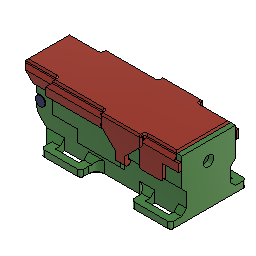
ratcase 1 v10 (Autodesk Fusion 360 design; units mm, degrees)
Autodesk Fusion 360 part; units mm, degrees
sketch "Sketch1" plane through (0, 0, 0) normal (0, 0, 1) x (1, 0, 0)
  line L0 (38, -11) -> (-38, -11)
  line L1 (-38, -11) -> (-38, 11)
  line L2 (-38, 11) -> (38, 11)
  line L3 (38, 11) -> (38, -11)
  line L4 (38, -11) -> (-38, 11) construction
  line L5 (-38, -11) -> (38, 11) construction
  line L6 (41, -14) -> (-41, -14)
  line L7 (-41, -14) -> (-41, 14)
  line L8 (-41, 14) -> (41, 14)
  line L9 (41, 14) -> (41, -14)
  dimension "d1" = 76
  dimension "d2" = 22
  dimension "d3" = -3
  constraint horizontal L0
  constraint perpendicular L0 L1
  constraint parallel L0 L2
  constraint parallel L1 L3
  constraint coincident L4 origin
  constraint coincident L5 origin
  measures "d1" distance of L1.end L2.end
  measures "d2" distance of L0.end L1.end
extrude "Extrude1" add sketch "Sketch1" along normal blind 20 makes body 1
sketch "Sketch15" plane through (0, 0, 20) normal (0, 0, 1) x (-1, 0, 0)
  line L0 (38, -11) -> (-38, -11)
  line L1 (-38, -11) -> (-38, 11)
  line L2 (-38, 11) -> (38, 11)
  line L3 (38, 11) -> (38, -11)
  line L4 (-41, -14) -> (41, -14)
  line L5 (41, -14) -> (41, 14)
  line L6 (41, 14) -> (-41, 14)
  line L7 (-41, 14) -> (-41, -14)
  line L8 (38, -11) -> (39, -11)
  line L9 (39, -11) -> (39, -7)
  line L10 (39, -7) -> (38, -7)
  line L11 (38, -7) -> (38, -11)
  line L12 (-38, 11) -> (-39, 11)
  line L13 (-39, 11) -> (-39, 7)
  line L14 (-39, 7) -> (-38, 7)
  line L15 (-38, 7) -> (-38, 11)
  dimension "d64" = 1
  dimension "d65" = 4
  dimension "d66" = 1
  dimension "d67" = 4
  constraint horizontal L8
  constraint vertical L9
  constraint horizontal L10
  constraint vertical L11
  constraint coincident L0.start L3.end
  constraint horizontal L12
  constraint vertical L13
  constraint horizontal L14
  constraint vertical L15
  constraint coincident L1.end L2.start
  measures "d64" distance of L1.end L12.end
  measures "d65" distance of L12.end L13.end
  measures "d66" distance of L9.end L10.end
  measures "d67" distance of L8.end L9.end
extrude "Extrude15" cut sketch "Sketch15" against normal blind 59 contours L3 L8 L9 L10 L11 | L1 L12 L13 L14 L15 bodies 1
sketch "Sketch2" plane through (0, 0, 0) normal (0, 0, -1) x (1, 0, 0)
  line L0 (38, -11) -> (-39, -11)
  line L1 (-38, -7) -> (-38, 11)
  line L2 (-38, 11) -> (39, 11)
  line L3 (38, 7) -> (38, -11)
  line L4 (-41, -14) -> (41, -14)
  line L5 (41, -14) -> (41, 14)
  line L6 (41, 14) -> (-41, 14)
  line L7 (-41, 14) -> (-41, -14)
  line L8 (-41, 14) -> (41, 14)
  line L9 (41, 14) -> (41, -14)
  line L10 (41, -14) -> (-41, -14)
  line L11 (-41, -14) -> (-41, 14)
  line L12 (39, 7) -> (38, 7)
  line L13 (-39, -7) -> (-38, -7)
  line L14 (39, 11) -> (39, 7)
  line L15 (-39, -11) -> (-39, -7)
  constraint horizontal L8
  constraint vertical L9
  constraint horizontal L10
  constraint vertical L11
  constraint coincident L4.end L5.start
  constraint coincident L6.end L7.start
extrude "Extrude2" add sketch "Sketch2" along normal blind 3 contours L0 L1 L2 L3 L12 L13 L14 L15 | L4 L5 L6 L7 L8 L9 L10 L11 bodies 1
sketch "Sketch3" plane through (0, 0, 20) normal (0, 0, 1) x (-1, 0, 0)
  line L0 (-38, -11) -> (-38, 7)
  line L1 (-41, -14) -> (41, -14)
  line L2 (41, -14) -> (41, 14)
  line L3 (41, 14) -> (-41, 14)
  line L4 (-41, 14) -> (-41, -14)
  line L5 (38, -14) -> (-2, -14)
  line L6 (-2, -14) -> (-2, 14)
  line L7 (-2, 14) -> (38, 14)
  line L8 (38, 14) -> (38, -14)
  line L9 (38, -14) -> (-2, 14) construction
  line L10 (-2, -14) -> (38, 14) construction
  line L11 (18, 0) -> (0, 0) construction
  line L12 (-31, 14) -> (-7, 14)
  line L13 (-7, 14) -> (-7, -14)
  line L14 (-7, -14) -> (-31, -14)
  line L15 (-31, -14) -> (-31, 14)
  line L16 (-31, 14) -> (-7, -14) construction
  line L17 (-7, 14) -> (-31, -14) construction
  line L18 (0, 0) -> (-19, 0) construction
  line L19 (41, -17) -> (-41, -17)
  line L20 (-41, -17) -> (-41, 17)
  line L21 (-41, 17) -> (41, 17)
  line L22 (41, 17) -> (41, -17)
  line L23 (-38, 7) -> (-39, 7)
  line L24 (-39, 11) -> (38, 11)
  line L25 (38, 11) -> (38, -7)
  line L26 (38, -7) -> (39, -7)
  line L27 (39, -7) -> (39, -11)
  line L28 (39, -11) -> (-38, -11)
  line L29 (-39, 7) -> (-39, 11)
  point P0 (18, 0)
  point P1 (-19, 0)
  dimension "d8" = 28
  dimension "d9" = 40
  dimension "d10" = 24
  dimension "d13" = 3
  dimension "d14" = 3
  dimension "d68" = 5
  constraint horizontal L5
  constraint perpendicular L5 L6
  constraint parallel L5 L7
  constraint parallel L6 L8
  constraint coincident L9 P0
  constraint coincident L10 P0
  constraint coincident P0 L11.start
  constraint coincident L11.end L18.start
  constraint horizontal L11
  constraint horizontal L12
  constraint perpendicular L12 L13
  constraint parallel L12 L14
  constraint parallel L13 L15
  constraint coincident L16 P1
  constraint coincident L17 P1
  constraint coincident P1 L18.end
  constraint parallel L11 L18
  constraint collinear L5 L14
  constraint horizontal L19
  constraint vertical L20
  constraint horizontal L21
  constraint vertical L22
  constraint collinear L2 L22
  constraint collinear L4 L20
  constraint collinear L8 L25
  measures "d8" distance of L5.start L7.end
  measures "d9" distance of L6.end L7.end
  measures "d10" distance of L12.start L12.end
  measures "d13" distance of L5 L19
  measures "d14" distance of L7 L21
  measures "d68" distance of L6 L13
extrude "Extrude3" add sketch "Sketch3" along normal blind 10 separate body contours L0 L1 L3 L4 L15 L20 L23 L24 L28 L29 | L1 L5 L14 L19 L20 L22 | L1 L6 L13 L28 | L3 L7 L12 L20 L21 L22 | L3 L6 L13 L24 | L1 L2 L3 L8 L22 L25 L26 L27 L28 makes body 2
sketch "Sketch10" plane through (41, 0, 0) normal (1, 0, 0) x (0, 1, 0)
  line L0 (14, -3) -> (14, 20)
  line L1 (14, 20) -> (-14, 20)
  line L2 (-14, 20) -> (-14, -3)
  line L3 (-14, -3) -> (14, -3)
  line L4 (-14, 20) -> (-17, 20)
  line L5 (-17, 20) -> (-17, 17)
  line L6 (-17, 17) -> (-14, 17)
  line L7 (-14, 17) -> (-14, 20)
  line L8 (14, 20) -> (17, 20)
  line L9 (17, 20) -> (17, 17)
  line L10 (17, 17) -> (14, 17)
  line L11 (14, 17) -> (14, 20)
  constraint horizontal L4
  constraint vertical L5
  constraint horizontal L6
  constraint vertical L7
  constraint coincident L1.end L2.start
  constraint horizontal L8
  constraint vertical L9
  constraint horizontal L10
  constraint vertical L11
  constraint coincident L0.end L1.start
extrude "Extrude10" add sketch "Sketch10" against normal up to surface (82 mm away) contours L0 L8 L9 L10 L11 | L2 L4 L5 L6 L7 bodies 1 2
sketch "Sketch4" plane through (0, 0, 20) normal (0, 0, 1) x (-1, 0, 0)
  line L0 (-2, 11) -> (38, 11)
  line L1 (22, -14) -> (22, 14)
  line L2 (1, -14) -> (1, 14)
  line L3 (38, -11) -> (38, -14)
  line L4 (38, 11) -> (38, 14)
  line L5 (-2, 14) -> (-2, 11)
  line L6 (38, 14) -> (-2, 14)
  line L7 (22, -14) -> (1, -14)
  line L8 (1, 14) -> (22, 14)
  line L9 (-2, -14) -> (-2, -11)
  dimension "d18" = 21
  dimension "d158" = 3
  constraint perpendicular L0 L1
  measures "d18" distance of L1 L2
  measures "d158" distance of L2 L9
extrude "Extrude4" cut sketch "Sketch4" against normal blind 7.5 contours L0 L1 L2 L6 L8 | L0 L1 L2 L7 bodies 1
sketch "Sketch5" plane through (0, -14, 0) normal (0, -1, 0) x (1, 0, 0)
  line L0 (-41, 17) -> (-41, -3)
  line L1 (-41, -3) -> (41, -3)
  line L2 (41, -3) -> (41, 17)
  line L3 (-1, 12.5) -> (-22, 12.5)
  line L4 (-25, 20) -> (-25, 9.5)
  line L5 (-25, 9.5) -> (2, 9.5)
  line L6 (2, 9.5) -> (2, 20)
  line L7 (-25, 20) -> (2, 20)
  line L8 (-22, 17) -> (-41, 17)
  line L9 (41, 17) -> (-1, 17)
  line L10 (-1, 17) -> (-1, 12.5)
  line L11 (-22, 12.5) -> (-22, 17)
  dimension "d22" = 3
  dimension "d159" = 3
  dimension "d160" = 3
  constraint perpendicular L0 L5
  constraint vertical L4
  measures "d22" distance of L3 L5
  measures "d159" distance of L4 L11
  measures "d160" distance of L6 L10
extrude "Extrude5" add sketch "Sketch5" along normal blind 3 contours L3 L4 L5 L6 L8 L9 L10 L11 | L3 L4 L6 L7 L8 L9 L10 L11 bodies 1
sketch "Sketch16" plane through (0, 14, 0) normal (0, 1, 0) x (-1, 0, 0)
  line L0 (1, 17) -> (-41, 17)
  line L1 (-41, 17) -> (-41, -3)
  line L2 (-41, -3) -> (41, -3)
  line L3 (41, -3) -> (41, 17)
  line L4 (-2, 17) -> (25, 17)
  line L5 (25, 17) -> (25, 9.5)
  line L6 (25, 9.5) -> (-2, 9.5)
  line L7 (-2, 9.5) -> (-2, 17)
  line L8 (22, 12.5) -> (1, 12.5)
  line L9 (22, 17) -> (22, 12.5)
  line L10 (22, 12.5) -> (1, 12.5)
  line L11 (1, 12.5) -> (1, 17)
  line L12 (41, 17) -> (22, 17)
  dimension "d60" = 3
  dimension "d69" = 3
  dimension "d70" = 3
  constraint horizontal L4
  constraint vertical L5
  constraint horizontal L6
  constraint vertical L7
  constraint coincident L0 L4.start
  measures "d60" distance of L6 L8
  measures "d69" distance of L7 L11
  measures "d70" distance of L5 L9
extrude "Extrude16" add sketch "Sketch16" along normal up to surface (3 mm away) contours L0 L4 L5 L6 L7 L8 L9 L10 L11 L12 | L4 L8 L9 L10 L11 bodies 1
sketch "Sketch7" plane through (41, 0, 0) normal (1, 0, 0) x (0, 1, 0)
  line L0 (14, -3) -> (14, 17)
  line L1 (17, 17) -> (17, 30)
  line L2 (17, 30) -> (-17, 30)
  line L3 (-14, 17) -> (-14, -3)
  line L4 (-14, -3) -> (14, -3)
  circle A0 centre (0, 24) radius 3.25
  line L5 (14, 17) -> (17, 17)
  line L6 (-17, 30) -> (-17, 17)
  line L7 (-17, 17) -> (-14, 17)
  dimension "d28" = 6.5
  dimension "d29" = 6
  measures "d28" diameter of A0
  measures "d29" distance of L2 A0.centre
extrude "Extrude7" cut sketch "Sketch7" against normal blind 6 contours A0 bodies 1
sketch "Sketch8" plane through (0, 0, 30) normal (0, 0, 1) x (-1, 0, 0)
  line L0 (-7, -14) -> (-31, -14)
  line L1 (-31, -14) -> (-31, -11)
  line L2 (-31, 14) -> (-7, 14)
  line L3 (38, 14) -> (38, -7)
  line L4 (41, 17) -> (-41, 17)
  line L5 (-41, 17) -> (-41, -17)
  line L6 (-41, -17) -> (41, -17)
  line L7 (41, -17) -> (41, 17)
  line L8 (-7, 11) -> (-4, 11)
  line L9 (-4, 11) -> (-4, 14)
  line L10 (-4, 14) -> (-7, 14)
  line L11 (-7, 14) -> (-7, 11)
  line L12 (-7, 14) -> (-7, 11)
  line L13 (-2, 11) -> (-2, 14)
  line L14 (-2, 14) -> (38, 14)
  line L15 (38, -14) -> (-2, -14)
  line L16 (-38, 7) -> (-39, 7)
  line L17 (-39, 7) -> (-39, 11)
  line L18 (-39, 11) -> (-31, 11)
  line L19 (-31, 11) -> (-31, 14)
  line L20 (-7, 11) -> (-2, 11)
  line L21 (38, -7) -> (39, -7)
  line L22 (39, -7) -> (39, -11)
  line L23 (39, -11) -> (38, -11)
  line L24 (38, -11) -> (38, -14)
  line L25 (-2, -14) -> (-2, -11)
  line L26 (-2, -11) -> (-7, -11)
  line L27 (-7, -11) -> (-7, -14)
  line L28 (-31, -11) -> (-38, -11)
  line L29 (-38, -11) -> (-38, 7)
  dimension "d71" = 3
  constraint horizontal L8
  constraint vertical L9
  constraint horizontal L10
  constraint vertical L11
  constraint coincident L2.end L10.end
  measures "d71" distance of L9.end L2.end
extrude "Extrude8" cut sketch "Sketch8" against normal up to surface (10 mm away) contours L8 L9 L10 L11 L12 L20 bodies 1
sketch "Sketch9" plane through (0, 0, 30) normal (0, 0, 1) x (-1, 0, 0)
  line L0 (38, 14) -> (38, -7)
  line L1 (-7, -14) -> (-31, -14)
  line L2 (-31, -14) -> (-31, -11)
  line L3 (-31, 14) -> (-4, 14)
  line L4 (41, 17) -> (-41, 17)
  line L5 (-41, 17) -> (-41, -17)
  line L6 (-41, -17) -> (41, -17)
  line L7 (41, -17) -> (41, 17)
  line L8 (-27.5, 14) -> (-19.5, 14)
  line L9 (-19.5, 14) -> (-19.5, 15)
  line L10 (-19.5, 15) -> (-27.5, 15)
  line L11 (-27.5, 15) -> (-27.5, 14)
  line L12 (-2, 11) -> (-2, 14)
  line L13 (-2, 14) -> (38, 14)
  line L14 (38, -14) -> (-2, -14)
  line L15 (-4, 14) -> (-4, 11)
  line L16 (-4, 11) -> (-2, 11)
  line L17 (38, -7) -> (39, -7)
  line L18 (39, -7) -> (39, -11)
  line L19 (39, -11) -> (38, -11)
  line L20 (38, -11) -> (38, -14)
  line L21 (-2, -14) -> (-2, -11)
  line L22 (-2, -11) -> (-7, -11)
  line L23 (-7, -11) -> (-7, -14)
  line L24 (-31, -11) -> (-38, -11)
  line L25 (-38, -11) -> (-38, 7)
  line L26 (-38, 7) -> (-39, 7)
  line L27 (-39, 7) -> (-39, 11)
  line L28 (-39, 11) -> (-31, 11)
  line L29 (-31, 11) -> (-31, 14)
  dimension "d35" = 8
  dimension "d36" = 1
  dimension "d72" = 3.5
  constraint horizontal L8
  constraint vertical L9
  constraint horizontal L10
  constraint vertical L11
  constraint coincident L3 L8.start
  measures "d35" distance of L9.end L10.end
  measures "d36" distance of L8.end L9.end
  measures "d72" distance of L11 L29
extrude "Extrude9" cut sketch "Sketch9" against normal up to surface (10 mm away) contours L3 L8 L9 L10 L11 bodies 1
sketch "Sketch11" plane through (41, 0, 0) normal (1, 0, 0) x (0, 1, 0)
  circle A0 centre (0, 24) radius 3.25
  line L0 (14, 17) -> (17, 17)
  line L1 (17, 17) -> (17, 30)
  line L2 (17, 30) -> (-17, 30)
  line L3 (-17, 30) -> (-17, 17)
  line L4 (-17, 17) -> (-14, 17)
  line L5 (-14, 17) -> (-14, -3)
  line L6 (-14, -3) -> (14, -3)
  line L7 (14, -3) -> (14, 17)
  line L8 (-17, 30) -> (17, 30)
  line L9 (17, 30) -> (17, 35)
  line L10 (17, 35) -> (-17, 35)
  line L11 (-17, 35) -> (-17, 30)
  dimension "d45" = 5
  constraint horizontal L8
  constraint vertical L9
  constraint horizontal L10
  constraint vertical L11
  constraint coincident L2.end L3.start
  measures "d45" distance of L2.end L10.end
extrude "Extrude11" add sketch "Sketch11" against normal up to surface (3 mm away) contours L2 L8 L9 L10 L11 bodies 1
sketch "Sketch12" plane through (0, 17, 0) normal (0, 1, 0) x (-1, 0, 0)
  line L0 (41, 17) -> (41, 30)
  line L1 (41, 30) -> (-38, 30)
  line L2 (-41, 35) -> (-41, 17)
  line L3 (-41, 17) -> (-2, 17)
  line L4 (-38, 30) -> (-39, 30)
  line L5 (-39, 30) -> (-39, 32.5)
  line L6 (-39, 32.5) -> (-38, 33.5)
  line L7 (-2, 17) -> (-2, 9.5)
  line L8 (-2, 9.5) -> (25, 9.5)
  line L9 (25, 9.5) -> (25, 17)
  line L10 (25, 17) -> (41, 17)
  line L11 (-38, 30) -> (-38, 35)
  line L12 (-38, 35) -> (-41, 35)
  line L13 (-38, 30) -> (-38, 33.5)
  constraint coincident L1.end L4.start
  constraint perpendicular L1 L5
extrude "Extrude12" cut sketch "Sketch12" against normal blind 34 contours L4 L5 L6 L11 L13 bodies 1
sketch "Sketch13" plane through (0, -17, 0) normal (0, -1, 0) x (1, 0, 0)
  line L0 (39, 30) -> (-41, 30)
  line L1 (-41, 30) -> (-41, 17)
  line L2 (-25, 9.5) -> (2, 9.5)
  line L3 (2, 9.5) -> (2, 17)
  line L4 (41, 17) -> (41, 35)
  line L5 (38, 30) -> (39, 30)
  line L6 (39, 30) -> (39, 33.5)
  line L7 (39, 33.5) -> (38, 33.5)
  line L8 (38, 33.5) -> (38, 30)
  line L9 (38, 33.5) -> (39, 32.5)
  line L10 (39, 32.5) -> (39, 30)
  line L11 (-41, 17) -> (-25, 17)
  line L12 (41, 35) -> (38, 35)
  line L13 (38, 35) -> (38, 33.5)
  line L14 (39, 32.5) -> (39, 30)
  line L15 (-25, 17) -> (-25, 9.5)
  line L16 (2, 17) -> (41, 17)
  constraint horizontal L5
  constraint vertical L6
  constraint horizontal L7
  constraint vertical L8
  constraint coincident L0 L5.start
  constraint coincident L0.start L5.end
  constraint coincident L7.end L8.start
  constraint coincident L9.end L10.start
extrude "Extrude13" add sketch "Sketch13" against normal blind 3 contours L0 L5 L6 L8 L9 L10 L14 bodies 1
sketch "Sketch14" plane through (0, 17, 0) normal (0, 1, 0) x (-1, 0, 0)
  line L0 (41, 30) -> (-39, 30)
  line L1 (-41, 35) -> (-41, 17)
  line L2 (-41, 17) -> (-2, 17)
  line L3 (41, 17) -> (41, 30)
  line L4 (-39, 30) -> (-38, 30)
  line L5 (-38, 30) -> (-38, 33.5)
  line L6 (-38, 33.5) -> (-39, 33.5)
  line L7 (-39, 33.5) -> (-39, 30)
  line L8 (-2, 17) -> (-2, 9.5)
  line L9 (-2, 9.5) -> (25, 9.5)
  line L10 (25, 9.5) -> (25, 17)
  line L11 (25, 17) -> (41, 17)
  line L12 (-39, 32.5) -> (-38, 33.5)
  line L13 (-38, 33.5) -> (-38, 35)
  line L14 (-38, 35) -> (-41, 35)
  line L15 (-39, 30) -> (-39, 32.5)
  line L16 (-39, 32.5) -> (-39, 30)
  constraint horizontal L4
  constraint vertical L5
  constraint horizontal L6
  constraint vertical L7
  constraint coincident L0.end L4.start
  constraint coincident L12.start L15.end
extrude "Extrude14" add sketch "Sketch14" against normal blind 3 contours L0 L4 L5 L7 L12 L15 L16 bodies 1
chamfer "Chamfer1" distance 3 angle 45 2 edges at (-33, 14, 17) (21.5, 14, 17) on bodies 1
chamfer "Chamfer1" distance 3 angle 45 1 edges at (-11.5, 14, 9.5) on bodies 1
chamfer "Chamfer2" distance 3 angle 45 3 edges at (-33, -14, 17) (-11.5, -14, 9.5) (21.5, -14, 17) on bodies 1
sketch "Sketch17" plane through (0, 0, -3) normal (0, 0, -1) x (1, 0, 0)
  line L0 (-41, -14) -> (41, -14)
  line L1 (41, -14) -> (41, 14)
  line L2 (41, 14) -> (-41, 14)
  line L3 (-41, 14) -> (-41, -14)
  line L4 (41, 14) -> (16, 14)
  line L5 (16, 14) -> (16, 24)
  line L6 (16, 24) -> (41, 24)
  line L7 (41, 24) -> (41, 14)
  line L8 (21, 14) -> (36, 14)
  line L9 (36, 14) -> (36, 19)
  line L10 (36, 19) -> (21, 19)
  line L11 (21, 19) -> (21, 14)
  line L12 (-41, 14) -> (-16, 14)
  line L13 (-16, 14) -> (-16, 24)
  line L14 (-16, 24) -> (-41, 24)
  line L15 (-41, 24) -> (-41, 14)
  line L16 (-36, 14) -> (-21, 14)
  line L17 (-21, 14) -> (-21, 19)
  line L18 (-21, 19) -> (-36, 19)
  line L19 (-36, 19) -> (-36, 14)
  line L20 (-41, -14) -> (-16, -14)
  line L21 (-16, -14) -> (-16, -24)
  line L22 (-16, -24) -> (-41, -24)
  line L23 (-41, -24) -> (-41, -14)
  line L24 (-36, -14) -> (-21, -14)
  line L25 (-21, -14) -> (-21, -19)
  line L26 (-21, -19) -> (-36, -19)
  line L27 (-36, -19) -> (-36, -14)
  line L28 (16, -14) -> (41, -14)
  line L29 (41, -14) -> (41, -24)
  line L30 (41, -24) -> (16, -24)
  line L31 (16, -24) -> (16, -14)
  line L32 (21, -14) -> (36, -14)
  line L33 (36, -14) -> (36, -19)
  line L34 (36, -19) -> (21, -19)
  line L35 (21, -19) -> (21, -14)
  point P0 (-41, -17)
  point P1 (41, -17)
  dimension "d73" = 5
  dimension "d74" = 5
  dimension "d75" = 5
  dimension "d76" = 5
  dimension "d77" = 15
  dimension "d78" = 5
  dimension "d79" = 10
  constraint horizontal L4
  constraint vertical L5
  constraint horizontal L6
  constraint vertical L7
  constraint coincident L1.end L2.start
  constraint horizontal L8
  constraint vertical L9
  constraint horizontal L10
  constraint vertical L11
  constraint coincident L2 L8.start
  constraint horizontal L12
  constraint vertical L13
  constraint horizontal L14
  constraint vertical L15
  constraint coincident L2.end L3.start
  constraint horizontal L16
  constraint vertical L17
  constraint horizontal L18
  constraint vertical L19
  constraint coincident L2 L16.start
  constraint horizontal L20
  constraint vertical L21
  constraint horizontal L22
  constraint vertical L23
  constraint horizontal L24
  constraint vertical L25
  constraint horizontal L26
  constraint vertical L27
  constraint coincident L20 L24.start
  constraint horizontal L28
  constraint vertical L29
  constraint horizontal L30
  constraint vertical L31
  constraint horizontal L32
  constraint vertical L33
  constraint horizontal L34
  constraint vertical L35
  constraint collinear L6 L14
  constraint collinear L22 L30
  constraint collinear L11 L35
  constraint collinear L9 L33
  constraint collinear L17 L25
  constraint collinear L19 L27
  constraint collinear L10 L18
  constraint collinear L26 L34
  constraint equal L19 L27
  constraint equal L15 L23
  constraint equal L22 L30
  constraint collinear L5 L31
  constraint collinear L13 L21
  constraint coincident L0.start L3.end
  constraint coincident L0.end L1.start
  constraint coincident L28 L32.end
  measures "d73" distance of L15 L19
  measures "d74" distance of L13 L17
  measures "d75" distance of L5 L11
  measures "d76" distance of L7 L9
  measures "d77" distance of L9.end L10.end
  measures "d78" distance of L12 L18
  measures "d79" distance of L12 L14
extrude "Extrude17" add sketch "Sketch17" against normal blind 5 contours L0 L20 L21 L22 L23 L25 L26 L27 | L2 L12 L13 L14 L15 L17 L18 L19 | L0 L28 L29 L30 L31 L33 L34 L35 | L2 L4 L5 L6 L7 L9 L10 L11 bodies 1
chamfer "Chamfer3" distance 3 angle 45 8 edges at (-38.5, -14, 2) (-18.5, -14, 2) (18.5, -14, 2) (38.5, -14, 2) (-38.5, 14, 2) (-18.5, 14, 2) (18.5, 14, 2) (38.5, 14, 2) on bodies 1
fillet "Fillet1" radius 2 4 edges at (41, 24, -0.5) (16, 24, -0.5) (-16, 24, -0.5) (-41, 24, -0.5) on bodies 1
fillet "Fillet2" radius 5 2 edges at (16, 14, 1) (-16, 14, 1) on bodies 1
fillet "Fillet3" radius 2 4 edges at (-41, -24, -0.5) (-16, -24, -0.5) (16, -24, -0.5) (41, -24, -0.5) on bodies 1
fillet "Fillet4" radius 5 2 edges at (16, -14, 1) (-16, -14, 1) on bodies 1
chamfer "Chamfer4" distance 1 angle 45 1 faces at (-3.6667, 4.6667, -3) on bodies 1
chamfer "Chamfer5" distance 1 angle 45 4 edges at (28.5, 19, 2) (-28.5, 19, 2) (-28.5, -19, 2) (28.5, -19, 2) on bodies 1
sketch "Sketch18" plane through (-41, 0, 0) normal (-1, 0, 0) x (0, -1, 0)
  line L0 (-22, -2) -> (22, -2)
  line L1 (22, -2) -> (22, 2)
  line L2 (22, 2) -> (17, 2)
  line L3 (17, 2) -> (14, 5)
  line L4 (14, 5) -> (14, 14)
  line L5 (17, 17) -> (17, 30)
  line L6 (17, 30) -> (-17, 30)
  line L7 (-17, 30) -> (-17, 17)
  line L8 (-17, 17) -> (-14, 14)
  line L9 (-14, 14) -> (-14, 5)
  line L10 (-14, 5) -> (-17, 2)
  line L11 (-17, 2) -> (-22, 2)
  line L12 (-22, 2) -> (-22, -2)
  line L13 (-9, 9.5) -> (-9, 30)
  line L14 (0, 0) -> (0, 30)
  line L15 (9, 9.5) -> (9, 30)
  line L16 (-14, 9.5) -> (-9, 9.5)
  line L17 (9, 9.5) -> (14, 9.5)
  line L18 (-14, 14) -> (-14, 30)
  line L19 (14, 14) -> (14, 30)
  line L20 (14, 14) -> (17, 17)
  dimension "d93" = 8
  constraint coincident L6 L13.end
  constraint perpendicular L6 L13
  constraint coincident L14.start origin
  constraint midpoint L6 L14.end
  constraint symmetric L13.start L14 L15.start
  constraint symmetric L13.end L14 L15.end
  constraint midpoint L9 L16.start
  constraint perpendicular L13 L16
  constraint midpoint L4 L17.end
  constraint perpendicular L4 L17
  constraint coincident L8.end L9.start
  constraint coincident L6 L18.end
  constraint perpendicular L6 L18
  constraint coincident L4.end L19.start
  constraint coincident L6 L19.end
  constraint perpendicular L6 L19
  measures "d93" distance of L7 L13
extrude "Extrude18" add sketch "Sketch18" along normal blind 13 contours L6 L9 L13 L16 L18 | L4 L6 L15 L17 L19 bodies 1
sketch "Sketch2 (2)" plane through (0, 0, 0) normal (1, 0, 0) x (0, 1, 0) in component "cam mount"
  line L0 (-4.5, -4.5) -> (4.5, -4.5)
  line L1 (4.5, -4.5) -> (4.5, 4.5)
  line L2 (4.5, 4.5) -> (-4.5, 4.5)
  line L3 (-4.5, 4.5) -> (-4.5, -4.5)
  line L4 (-4.5, -4.5) -> (4.5, 4.5) construction
  line L5 (4.5, -4.5) -> (-4.5, 4.5) construction
  line L6 (8.5, 8.5) -> (-8.5, 8.5)
  line L7 (-8.5, 8.5) -> (-8.5, -8.5)
  line L8 (-8.5, -8.5) -> (8.5, -8.5)
  line L9 (8.5, -8.5) -> (8.5, 8.5)
  line L10 (-4.5, 4.5) -> (-4.5, 8.5)
  line L11 (4.5, 4.5) -> (4.5, 8.5)
  dimension "d96" = 9
  dimension "d97" = 9
  dimension "d98" = 4
  constraint horizontal L0
  constraint perpendicular L0 L1
  constraint parallel L0 L2
  constraint parallel L1 L3
  constraint coincident L4 origin
  constraint coincident L5 origin
  constraint coincident L6 L10.end
  constraint perpendicular L6 L10
  constraint coincident L6 L11.end
  constraint perpendicular L6 L11
  measures "d96" distance of L0.start L2.end
  measures "d97" distance of L0.start L0.end
extrude "Extrude1'" add sketch "Sketch2 (2)" along normal blind 8 separate body contours L0 L1 L3 L6 L7 L8 L9 L10 L11 makes body 3 in component "cam mount"
sketch "Sketch3 (2)" plane through (8, 0, 0) normal (1, 0, 0) x (0, 1, 0) in component "cam mount"
  line L0 (-4.5, -4.5) -> (-4.5, 8.5)
  line L1 (-4.5, 8.5) -> (-8.5, 8.5)
  line L2 (-8.5, 8.5) -> (-8.5, -8.5)
  line L3 (-8.5, -8.5) -> (8.5, -8.5)
  line L4 (8.5, -8.5) -> (8.5, 8.5)
  line L5 (8.5, 8.5) -> (4.5, 8.5)
  line L6 (4.5, 8.5) -> (4.5, -4.5)
  line L7 (4.5, -4.5) -> (-4.5, -4.5)
  line L8 (-8.5, -8.5) -> (8.5, -8.5)
  line L9 (8.5, -8.5) -> (8.5, 8.5)
  line L10 (8.5, 8.5) -> (-8.5, 8.5)
  line L11 (-8.5, 8.5) -> (-8.5, -8.5)
  constraint horizontal L8
  constraint vertical L9
  constraint horizontal L10
  constraint vertical L11
  constraint coincident L4.end L5.start
  constraint coincident L2.end L3.start
extrude "Extrude2'" add sketch "Sketch3 (2)" along normal blind 3 bodies 3 in component "cam mount"
sketch "Sketch4 (2)" plane through (0, -8.5, 0) normal (0, -1, 0) x (1, 0, 0) in component "cam mount"
  line L0 (0, 8.5) -> (0, -8.5)
  line L1 (0, -8.5) -> (11, -8.5)
  line L2 (11, -8.5) -> (11, 8.5)
  line L3 (11, 8.5) -> (0, 8.5)
  circle A0 centre (5, 0) radius 3
extrude "Extrude3'" add sketch "Sketch4 (2)" along normal blind 6 contours A0 bodies 3 in component "cam mount"
sketch "Sketch5 (2)" plane through (0, 8.5, 0) normal (0, 1, 0) x (-1, 0, 0) in component "cam mount"
  line L0 (0, -8.5) -> (0, 8.5)
  line L1 (0, 8.5) -> (-11, 8.5)
  line L2 (-11, 8.5) -> (-11, -8.5)
  line L3 (-11, -8.5) -> (0, -8.5)
  circle A0 centre (-5, 0) radius 3
  dimension "d105" = 6
  measures "d105" diameter of A0
extrude "Extrude4'" add sketch "Sketch5 (2)" along normal blind 6 contours A0 bodies 3 in component "cam mount"
sketch "Sketch19" plane through (0, -14, 0) normal (0, -1, 0) x (1, 0, 0)
  circle A0 centre (-51, 18) radius 3.05
  line L0 (-54, 21.05) -> (-51.7746, 20.95)
  line L1 (-54, 14.95) -> (-51.7746, 15.05)
  line L2 (-51.7746, 15.05) -> (-51.7746, 20.95)
  line L3 (-41, 9.5) -> (-54, 9.5)
  line L4 (-54, 14.95) -> (-54, 21.05)
  line L5 (-54, 21.05) -> (-51, 21.05) construction
  line L6 (-54, 9.5) -> (-54, 30)
  line L7 (-36, -2) -> (-21, -2)
  line L8 (-21, -2) -> (-21, 5)
  line L9 (-21, 5) -> (-11, 5)
  line L10 (-11, 5) -> (-11, -2)
  line L11 (-11, -2) -> (11, -2)
  line L12 (11, -2) -> (11, 5)
  line L13 (11, 5) -> (21, 5)
  line L14 (21, 5) -> (21, -2)
  line L15 (21, -2) -> (36, -2)
  line L16 (36, -2) -> (36, 5)
  line L17 (36, 5) -> (41, 5)
  line L18 (41, 5) -> (41, 14)
  line L19 (41, 14) -> (2, 14)
  line L20 (2, 14) -> (2, 6.5)
  line L21 (2, 6.5) -> (-25, 6.5)
  line L22 (-25, 6.5) -> (-25, 14)
  line L23 (-25, 14) -> (-41, 14)
  line L24 (-41, 14) -> (-41, 30)
  line L25 (-41, 30) -> (-54, 30)
  line L26 (-54, 30) -> (-54, 9.5)
  line L27 (-54, 9.5) -> (-41, 9.5)
  line L28 (-41, 9.5) -> (-41, 5)
  line L29 (-41, 5) -> (-36, 5)
  line L30 (-36, 5) -> (-36, -2)
  line L31 (-36, -2) -> (-21, -2)
  line L32 (-21, -2) -> (-21, 5)
  line L33 (-21, 5) -> (-11, 5)
  line L34 (-11, 5) -> (-11, -2)
  line L35 (-11, -2) -> (11, -2)
  line L36 (11, -2) -> (11, 5)
  line L37 (11, 5) -> (21, 5)
  line L38 (21, 5) -> (21, -2)
  line L39 (21, -2) -> (36, -2)
  line L40 (36, -2) -> (36, 5)
  line L41 (36, 5) -> (41, 5)
  line L42 (41, 5) -> (41, 14)
  line L43 (41, 14) -> (2, 14)
  line L44 (2, 14) -> (2, 6.5)
  line L45 (2, 6.5) -> (-25, 6.5)
  line L46 (-25, 6.5) -> (-25, 14)
  line L47 (-25, 14) -> (-41, 14)
  line L48 (-41, 14) -> (-41, 30)
  line L49 (-41, 30) -> (-54, 30)
  line L50 (-54, 30) -> (-54, 9.5)
  line L51 (-54, 9.5) -> (-41, 9.5)
  line L52 (-41, 9.5) -> (-41, 5)
  line L53 (-41, 5) -> (-36, 5)
  line L54 (-36, 5) -> (-36, -2)
  dimension "d108" = 0.1
  dimension "d111" = 0.1
  dimension "d112" = 6.1
  dimension "d151" = 8.5
  dimension "d161" = 3
  constraint coincident A0 L0.end
  constraint coincident A0 L1.end
  constraint vertical L2
  constraint coincident A0 L5.end
  constraint horizontal L5
  constraint tangent A0 L5
  constraint vertical L4
  constraint collinear L4 L6
  measures "d108" vertical distance of L0.start L0.end
  measures "d111" vertical distance of L1.start L1.end
  measures "d112" diameter of A0
  measures "d151" distance of A0.centre L3
  measures "d161" distance of A0.centre L4
extrude "Extrude19" cut sketch "Sketch19" against normal through all contours A0 L2 | A0 L2 L4 L6 L26 L50 | A0 L0 L4 L6 L26 L50 | A0 L1 L4 L6 L26 L50 | A0 L4 L6 L26 L50 bodies 1
fillet "Fillet1'" radius 2 4 edges at (5.5, -8.5, -8.5) (5.5, -8.5, 8.5) (5.5, 8.5, 8.5) (5.5, 8.5, -8.5) on bodies 3 in component "cam mount"
sketch "Sketch1 (2)" plane through (0, 0, 30) normal (0, 0, 1) x (-1, 0, 0) in component "lid"
  line L0 (-38, -14) -> (-38, -17)
  line L1 (-38, -17) -> (41, -17)
  line L2 (41, 17) -> (-38, 17)
  line L3 (-38, 17) -> (-38, 14)
  line L4 (-38, 14) -> (-39, 14)
  line L5 (-39, 14) -> (-39, 11)
  line L6 (-39, 11) -> (-31, 11)
  line L7 (-31, 11) -> (-31, 14)
  line L8 (-31, 14) -> (-27.5, 14)
  line L9 (-27.5, 14) -> (-27.5, 15)
  line L10 (-27.5, 15) -> (-19.5, 15)
  line L11 (-19.5, 15) -> (-19.5, 14)
  line L12 (-19.5, 14) -> (-4, 14)
  line L13 (-4, 14) -> (-4, 11)
  line L14 (-4, 11) -> (-2, 11)
  line L15 (-2, 11) -> (-2, 14)
  line L16 (-2, 14) -> (38, 14)
  line L17 (38, 14) -> (38, -7)
  line L18 (38, -7) -> (39, -7)
  line L19 (39, -7) -> (39, -11)
  line L20 (39, -11) -> (38, -11)
  line L21 (38, -11) -> (38, -14)
  line L22 (38, -14) -> (-2, -14)
  line L23 (-2, -14) -> (-2, -11)
  line L24 (-2, -11) -> (-7, -11)
  line L25 (-7, -11) -> (-7, -14)
  line L26 (-7, -14) -> (-31, -14)
  line L27 (-31, -14) -> (-31, -11)
  line L28 (-31, -11) -> (-38, -11)
  line L29 (-38, 7) -> (-39, 7)
  line L30 (-39, -14) -> (-38, -14)
  line L31 (54, -14) -> (54, -9)
  line L32 (40.9633, 11.0655) -> (41, 5.0657)
  line L33 (41, 5.0657) -> (38, 5.0657)
  line L34 (38, 11) -> (38, 5.0657)
  line L35 (38, 11) -> (-36.2027, 11)
  line L36 (-36.2027, 11) -> (-36.2027, -11)
  line L37 (-36.2027, -11) -> (38, -11)
  line L38 (38, -11) -> (38, -5)
  line L39 (38, -5) -> (41.0181, -5.0137)
  line L40 (-38, -17) -> (-38, -14)
  line L41 (-38, -14) -> (-39, -14)
  line L42 (-39, 14) -> (-38, 14)
  line L43 (-38, 14) -> (-38, 17)
  line L44 (41, -17) -> (41, -14)
  line L45 (-38, -11) -> (-38, 7)
  line L46 (-39, 7) -> (-39, -14)
  line L47 (-38, 17) -> (41, 17)
  line L48 (41, 14) -> (54, 14)
  line L49 (41, 17) -> (41, 14)
  line L50 (54, 14) -> (54, 9)
  line L51 (54, 9) -> (41, 9)
  line L52 (41, 9) -> (41, 5.0657)
  line L53 (41, -9) -> (41.0181, -5.0137)
  line L54 (41, -14) -> (41, -17)
  line L55 (-38, -17) -> (41, -17)
  line L56 (41, -14) -> (54, -14)
  line L57 (54, -14) -> (54, -9)
  line L58 (54, -9) -> (41, -9)
  line L59 (41, 9) -> (54, 9)
  line L60 (54, 9) -> (54, 14)
  line L61 (54, 14) -> (41, 14)
  line L62 (41, 14) -> (41, 17)
  line L63 (-39, 14) -> (-39, 7)
  line L64 (-39, 7) -> (-39, -14)
  dimension "d120" = 6
  dimension "d121" = 6
  constraint coincident L17 L33.end
  constraint perpendicular L17 L33
  constraint coincident L6 L35.end
  constraint coincident L17 L34.start
  constraint parallel L17 L34
  constraint coincident L28 L36.end
  constraint perpendicular L28 L36
  constraint coincident L20.end L21.start
  constraint perpendicular L20 L38
  constraint coincident L0.end L1.start
  constraint coincident L0.start L30.end
  constraint coincident L30.start L41.end
  constraint coincident L4.end L5.start
  constraint coincident L3.end L4.start
  constraint coincident L2.end L3.start
  constraint coincident L2.start L47.end
  constraint perpendicular L33 L52
  constraint perpendicular L39 L53
  constraint coincident L44.end L54.start
  constraint coincident L1.end L44.start
  constraint coincident L29.end L46.start
  measures "d120" distance of L32.start L32.end
  measures "d121" distance of L20.end L38.end
extrude "Extrude1''" add sketch "Sketch1 (2)" along normal blind 3 separate body contours L0 L1 L17 L18 L19 L20 L21 L22 L23 L24 L25 L26 L27 L28 L29 L30 L31 L37 L38 L39 L40 L41 L44 L45 L46 L53 L54 L55 L56 L57 L58 L64 | L6 L28 L29 L36 L45 L63 | L2 L3 L4 L5 L6 L7 L8 L9 L10 L11 L12 L13 L14 L15 L16 L17 L33 L34 L35 L42 L43 L47 L48 L49 L50 L51 L52 L59 L60 L61 L62 L63 makes body 4 in component "lid"
sketch "Sketch2 (3)" plane through (0, 0, 33) normal (0, 0, 1) x (-1, 0, 0) in component "lid"
  line L0 (-39, -14) -> (-38, -14)
  line L1 (-38, -14) -> (-38, -17)
  line L2 (-38, -17) -> (41, -17)
  line L3 (38, -5) -> (38, -7)
  line L4 (38, -7) -> (39, -7)
  line L5 (39, -7) -> (39, -11)
  line L6 (39, -11) -> (38, -11)
  line L7 (38, -11) -> (38, -14)
  line L8 (38, -14) -> (-2, -14)
  line L9 (-2, -14) -> (-2, -11)
  line L10 (-2, -11) -> (-7, -11)
  line L11 (-7, -11) -> (-7, -14)
  line L12 (-7, -14) -> (-31, -14)
  line L13 (-31, -14) -> (-31, -11)
  line L14 (-31, -11) -> (-36.2027, -11)
  line L15 (-36.2027, -11) -> (-36.2027, 11)
  line L16 (-36.2027, 11) -> (-31, 11)
  line L17 (-31, 11) -> (-31, 14)
  line L18 (-31, 14) -> (-27.5, 14)
  line L19 (41, 17) -> (-38, 17)
  line L20 (-38, 17) -> (-38, 14)
  line L21 (-38, 14) -> (-39, 14)
  line L22 (-38, 17) -> (41, 17)
  line L23 (41, -17) -> (-38, -17)
  line L24 (-38, -17) -> (-38, 17)
  line L25 (-39, 14) -> (-39, 7)
  line L26 (41, -17) -> (41, -14)
  line L27 (41.0181, -5.0137) -> (38, -5)
  line L28 (-27.5, 14) -> (-27.5, 15)
  line L29 (-27.5, 15) -> (-19.5, 15)
  line L30 (-19.5, 15) -> (-19.5, 14)
  line L31 (-19.5, 14) -> (-4, 14)
  line L32 (-4, 14) -> (-4, 11)
  line L33 (-4, 11) -> (-2, 11)
  line L34 (-2, 11) -> (-2, 14)
  line L35 (-2, 14) -> (38, 14)
  line L36 (38, 14) -> (38, 5.0657)
  line L37 (38, 5.0657) -> (41, 5.0657)
  line L38 (41, 14) -> (41, 17)
  line L39 (41, -14) -> (54, -14)
  line L40 (54, 14) -> (54, -14)
  line L41 (54, 14) -> (41, 14)
  line L42 (41, 5.0657) -> (41, 9)
  line L43 (41, 9) -> (54, 9)
  line L44 (54, 9) -> (54, 14)
  line L45 (54, 14) -> (41, 14)
  line L46 (41, -14) -> (54, -14)
  line L47 (54, -14) -> (54, -9)
  line L48 (54, -9) -> (41, -9)
  line L49 (41, -9) -> (41.0181, -5.0137)
  line L50 (-39, 7) -> (-39, -14)
  constraint horizontal L22
  constraint horizontal L23
  constraint vertical L24
  constraint coincident L2 L23.start
  constraint coincident L19.end L20.start
  constraint coincident L26.end L39.start
  constraint coincident L38.start L41.end
  constraint coincident L19.start L22.end
  constraint coincident L40.start L41.start
  constraint coincident L39.end L40.end
extrude "Extrude2''" add sketch "Sketch2 (3)" along normal blind 3 contours L1 L2 L3 L4 L5 L6 L7 L8 L9 L10 L11 L12 L13 L14 L15 L16 L17 L18 L19 L20 L22 L23 L24 L26 L27 L28 L29 L30 L31 L32 L33 L34 L35 L36 L37 L38 L39 L40 L41 L42 L43 L44 L45 L46 L47 L48 L49 | L3 L4 L5 L6 L7 L8 L9 L10 L11 L12 L13 L14 L15 L16 L17 L18 L27 L28 L29 L30 L31 L32 L33 L34 L35 L36 L37 L40 L42 L43 L48 L49 bodies 4 in component "lid"
sketch "Sketch4 (3)" plane through (0, -17, 0) normal (0, -1, 0) x (1, 0, 0) in component "lid"
  line L0 (38, 30) -> (38, 36)
  line L1 (2, 20) -> (2, 14)
  line L2 (2, 14) -> (8, 14)
  line L3 (8, 14) -> (8, 20)
  line L4 (8, 20) -> (18, 30)
  line L5 (18, 36) -> (-8, 36)
  line L6 (-8, 30) -> (2, 20)
  line L7 (-8, 30) -> (-8, 36)
  line L8 (18, 30) -> (18, 36)
  line L9 (38, 36) -> (-41, 36)
  line L10 (-41, 30) -> (38, 30)
  line L11 (-41, 36) -> (-41, 30)
  dimension "d137" = 6
  dimension "d138" = 6
  dimension "d176" = 45
  dimension "d178" = 45
  constraint vertical L1
  constraint perpendicular L1 L2
  constraint perpendicular L2 L3
  constraint vertical L7
  constraint equal L1 L3
  constraint vertical L8
  constraint coincident L4.end L10
  constraint coincident L6.start L10
  measures "d137" distance of L2.end L3.end
  measures "d138" distance of L1.end L2.end
  measures "d176" angle of L6 L7
  measures "d178" angle of L4 L10
sketch "Sketch7 (2)" plane through (0, 0, 30) normal (0, 0, -1) x (1, 0, 0) in component "lid"
  line L0 (36.2027, 11) -> (36.2027, -11)
  line L1 (36.2027, -11) -> (31, -11)
  line L2 (31, -11) -> (31, -14)
  line L3 (31, -14) -> (7, -14)
  line L4 (7, -14) -> (7, -11)
  line L5 (7, -11) -> (2, -11)
  line L6 (2, -11) -> (2, -14)
  line L7 (2, -14) -> (-38, -14)
  line L8 (-38, -14) -> (-38, -11)
  line L9 (-38, -11) -> (-39, -11)
  line L10 (-39, -11) -> (-39, -7)
  line L11 (-39, -7) -> (-38, -7)
  line L12 (-38, -7) -> (-38, -5)
  line L13 (-38, -5) -> (-41.0181, -5.0137)
  line L14 (-41.0181, -5.0137) -> (-41, -9)
  line L15 (-41, -9) -> (-54, -9)
  line L16 (-54, -9) -> (-54, -14)
  line L17 (-54, -14) -> (-41, -14)
  line L18 (-41, -14) -> (-41, -17)
  line L19 (-41, -17) -> (38, -17)
  line L20 (38, -17) -> (38, -14)
  line L21 (38, -14) -> (39, -14)
  line L22 (39, 7) -> (39, 14)
  line L23 (39, 14) -> (38, 14)
  line L24 (38, 14) -> (38, 17)
  line L25 (38, 17) -> (-41, 17)
  line L26 (-41, 17) -> (-41, 14)
  line L27 (-41, 14) -> (-54, 14)
  line L28 (-54, 14) -> (-54, 9)
  line L29 (-54, 9) -> (-41, 9)
  line L30 (-41, 9) -> (-41, 5.0657)
  line L31 (-41, 5.0657) -> (-38, 5.0657)
  line L32 (-38, 5.0657) -> (-38, 14)
  line L33 (-38, 14) -> (2, 14)
  line L34 (2, 14) -> (2, 11)
  line L35 (2, 11) -> (4, 11)
  line L36 (4, 11) -> (4, 14)
  line L37 (4, 14) -> (19.5, 14)
  line L38 (19.5, 14) -> (19.5, 15)
  line L39 (19.5, 15) -> (27.5, 15)
  line L40 (27.5, 15) -> (27.5, 14)
  line L41 (27.5, 14) -> (31, 14)
  line L42 (31, 14) -> (31, 11)
  line L43 (31, 11) -> (36.2027, 11)
  line L44 (38, 19) -> (-43, 19)
  line L45 (-43, 19) -> (-43, 16)
  line L46 (-43, 16) -> (-54, 16)
  line L47 (-54, -16) -> (-43, -16)
  line L48 (-43, -16) -> (-43, -19)
  line L49 (-43, -19) -> (38, -19)
  line L50 (38, -19) -> (41, -19)
  line L51 (41, -19) -> (41, -17)
  line L52 (41, -17) -> (38, -17)
  line L53 (-54, -16) -> (-54, -14)
  line L54 (-54, 14) -> (-54, 16)
  line L55 (38, 19) -> (41, 19)
  line L56 (41, 19) -> (41, 17)
  line L57 (38, 17) -> (41, 17)
  line L58 (39, -14) -> (39, 7)
  dimension "d162" = 2
  dimension "d163" = 2
  constraint perpendicular L20 L50
  constraint perpendicular L50 L51
  constraint coincident L19.end L20.start
  constraint perpendicular L20 L52
  constraint coincident L16.end L17.start
  constraint perpendicular L17 L53
  constraint coincident L27.end L28.start
  constraint perpendicular L46 L54
  constraint perpendicular L54 L55
  constraint perpendicular L55 L56
  constraint coincident L24.end L25.start
extrude "Extrude7'" add sketch "Sketch7 (2)" along normal blind 3 and the other way blind 2 contours L25 L26 L27 L44 L45 L46 L54 L55 L56 L57 | L17 L18 L19 L47 L48 L49 L50 L51 L52 L53 bodies 4 in component "lid"
sketch "Sketch8 (2)" plane through (0, 0, 27) normal (0, 0, -1) x (1, 0, 0) in component "lid"
  line L0 (-41, 17) -> (38, 17)
  line L1 (38, 17) -> (41, 17)
  line L2 (41, 17) -> (41, 19)
  line L3 (41, 19) -> (-43, 19)
  line L4 (-43, 19) -> (-43, 16)
  line L5 (-43, 16) -> (-54, 16)
  line L6 (-54, 16) -> (-54, 14)
  line L7 (-54, 14) -> (-41, 14)
  line L8 (-41, 14) -> (-41, 17)
  line L9 (-54, 14.4) -> (-41.4, 14.4)
  line L10 (-41.4, 14.4) -> (-41.4, 17.4)
  line L11 (-41.4, 17.4) -> (38, 17.4)
  line L12 (38, 17.4) -> (41, 17.4)
  dimension "d168" = -0.4
  constraint coincident L2 L12.end
  constraint perpendicular L2 L12
extrude "Extrude8'" cut sketch "Sketch8 (2)" against normal blind 3 contours L0 L1 L2 L6 L7 L8 L9 L10 L11 L12 bodies 4 in component "lid"
sketch "Sketch9 (2)" plane through (0, 0, 27) normal (0, 0, -1) x (1, 0, 0) in component "lid"
  line L0 (-43, -16) -> (-43, -19)
  line L1 (-43, -19) -> (41, -19)
  line L2 (41, -19) -> (41, -17)
  line L3 (41, -17) -> (-41, -17)
  line L4 (-41, -17) -> (-41, -14)
  line L5 (-41, -14) -> (-54, -14)
  line L6 (-54, -14) -> (-54, -16)
  line L7 (-54, -16) -> (-43, -16)
  line L8 (41, -17.4) -> (-41.4, -17.4)
  line L9 (-41.4, -17.4) -> (-41.4, -14.4)
  line L10 (-41.4, -14.4) -> (-54, -14.4)
  dimension "d171" = -0.4
extrude "Extrude9'" cut sketch "Sketch9 (2)" against normal blind 3 contours L2 L3 L4 L5 L6 L8 L9 L10 bodies 4 in component "lid"
chamfer "Chamfer7" distance 2 angle 45 6 edges at (-47.5, -14, 32) (-41, -15.5, 32) (-1.5, -17, 32) (-47.5, 14, 32) (-41, 15.5, 32) (-1.5, 17, 32) on bodies 4 in component "lid"
extrude "Extrude5'" add sketch "Sketch4 (3)" along normal blind 3 contours L5 L7 L8 L9 L10 | L1 L2 L3 L4 L6 L10 bodies 4 in component "lid"
sketch "Sketch5 (3)" plane through (8, 0, 0) normal (1, 0, 0) x (0, 1, 0) in component "lid"
  line L0 (-17, 14) -> (-17, 20)
  line L1 (-17, 20) -> (-20, 20)
  line L2 (-20, 20) -> (-20, 14)
  line L3 (-20, 14) -> (-17, 14)
  line L4 (-17, 14) -> (-16.5, 14)
  line L5 (-16.5, 14) -> (-16.5, 16.5)
  line L6 (-16.5, 16.5) -> (-17, 17)
  dimension "d144" = 0.5
  dimension "d145" = 2.5
  constraint coincident L0.start L3.end
  constraint perpendicular L0 L4
  constraint perpendicular L4 L5
  constraint midpoint L0 L6.end
  measures "d144" distance of L0.start L4.end
  measures "d145" distance of L4.end L5.end
extrude "Extrude6" add sketch "Sketch5 (3)" against normal blind 6 contours L0 L4 L5 L6 bodies 4 in component "lid"
chamfer "Chamfer3'" distance 1 angle 45 1 edges at (5, -16.5, 14) on bodies 4 in component "lid"
chamfer "Chamfer4'" distance 1 angle 45 1 edges at (5, -20, 14) on bodies 4 in component "lid"
extrude "Extrude13'" add 1 faces at (-54, 3, 35) along direction (-1, 0, 0) blind 7 on bodies 4 bodies 4 in component "lid"
mirror "Mirror1" about plane through (0, 0, 0) normal (0, 1, 0) of "Extrude5'", "Extrude6", "Chamfer3'", "Chamfer4'" in component "lid"
fillet "Fillet2'" radius 1 10 edges at (-8, 20, 33) (-8, 17, 35) (18, 20, 33) (18, 17, 35) (18, -17, 35) (18, -20, 33) (-8, -20, 33) (-8, -17, 35) (-41, -14, 35) (-41, 14, 35) on bodies 4 in component "lid"
chamfer "Chamfer5'" distance 1 angle 45 1 faces at (-19.7643, -4.7643, 36) on bodies 4 in component "lid"
sketch "Sketch10 (2)" plane through (41, 0, 0) normal (1, 0, 0) x (0, 1, 0) in component "lid"
  line L0 (-17.4, 27) -> (-17.4, 30)
  line L1 (-17.4, 30) -> (-17, 30)
  line L2 (-17, 30) -> (-17, 32)
  line L3 (-17, 32) -> (-19, 32)
  line L4 (-19, 32) -> (-19, 27)
  line L5 (-19, 27) -> (-17.4, 27)
  line L6 (-17.4, 30) -> (-17, 30)
  line L7 (-17, 30) -> (-17, 17)
  line L8 (-17, 17) -> (-17.4, 17)
  line L9 (-17.4, 17) -> (-17.4, 30)
  line L10 (17.4, 30) -> (17, 30)
  line L11 (17, 30) -> (17, 17)
  line L12 (17, 17) -> (17.4, 17)
  line L13 (17.4, 17) -> (17.4, 30)
  point P0 (17.4, 30)
  point P1 (17, 17)
  point P2 (-17, 17)
  constraint horizontal L6
  constraint vertical L7
  constraint horizontal L8
  constraint vertical L9
  constraint coincident L0.end L1.start
  constraint horizontal L10
  constraint vertical L11
  constraint horizontal L12
  constraint vertical L13
  constraint coincident P0 L10.start
  constraint coincident P1 L11.end
  constraint coincident P2 L7.end
extrude "Extrude10'" cut sketch "Sketch10 (2)" against normal blind 62 contours L0 L1 L6 L7 L8 L9 | L10 L11 L12 L13 bodies 4 in component "lid"
sketch "Sketch6" plane through (0, 0, 0) normal (-1, 0, 0) x (0, -1, 0) in component "cam mount"
  arc A0 (-8.5, -6.5) -> (-6.5, -8.5) centre (-6.5, -6.5) ccw
  line L0 (-6.5, -8.5) -> (6.5, -8.5)
  arc A1 (6.5, -8.5) -> (8.5, -6.5) centre (6.5, -6.5) ccw
  line L1 (8.5, -6.5) -> (8.5, 6.5)
  arc A2 (8.5, 6.5) -> (6.5, 8.5) centre (6.5, 6.5) ccw
  line L2 (6.5, 8.5) -> (4.5, 8.5)
  line L3 (4.5, 8.5) -> (4.5, -4.5)
  line L4 (4.5, -4.5) -> (-4.5, -4.5)
  line L5 (-4.5, -4.5) -> (-4.5, 8.5)
  line L6 (-4.5, 8.5) -> (-6.5, 8.5)
  arc A3 (-6.5, 8.5) -> (-8.5, 6.5) centre (-6.5, 6.5) ccw
  line L7 (-8.5, 6.5) -> (-8.5, -6.5)
  circle A4 centre (0, 0) radius 5.5
  dimension "d181" = 11
  constraint coincident A4.centre origin
  measures "d181" diameter of A4
extrude "Extrude5''" cut sketch "Sketch6" against normal blind 2.5 contours L5 A4 | L3 A4 | L4 A4 bodies 3 in component "cam mount"
extrude "Extrude6'" add 1 faces at (0, 7.4958, -0.1247) along direction (-1, 0, 0) blind 2.5 on bodies 3 bodies 3 in component "cam mount"
chamfer "Chamfer1'" distance 1 angle 45 1 faces at (11, 1.5, 2.1667) on bodies 3 in component "cam mount"
sketch "Sketch20" plane through (0, -17, 0) normal (0, -1, 0) x (1, 0, 0)
  line L0 (38, 30) -> (-41, 30)
  line L1 (-41, 30) -> (-41, 17)
  line L2 (-41, 17) -> (-25, 17)
  line L3 (-25, 17) -> (-25, 9.5)
  line L4 (-25, 9.5) -> (2, 9.5)
  line L5 (2, 9.5) -> (2, 17)
  line L6 (2, 17) -> (41, 17)
  line L7 (41, 17) -> (41, 35)
  line L8 (41, 35) -> (38, 35)
  line L9 (38, 35) -> (38, 30)
  line L10 (17.75, 27.75) -> (29.25, 27.75)
  line L11 (29.25, 27.75) -> (29.25, 18.25)
  line L12 (29.25, 18.25) -> (17.75, 18.25)
  line L13 (17.75, 18.25) -> (17.75, 27.75)
  line L14 (17.75, 23) -> (29.25, 23) construction
  line L15 (23.5, 23) -> (23.5, 27.75) construction
  line L16 (19.5, 30) -> (19.5, 20)
  line L17 (27.5, 20) -> (19.5, 20)
  dimension "d187" = 9.5
  dimension "d188" = 11.5
  dimension "d189" = 4
  dimension "d190" = 3
  constraint horizontal L10
  constraint vertical L11
  constraint horizontal L12
  constraint vertical L13
  constraint midpoint L13 L14.start
  constraint midpoint L11 L14.end
  constraint midpoint L14 L15.start
  constraint midpoint L10 L15.end
  measures "d187" distance of L10.start L12.end
  measures "d188" distance of L10.start L10.end
  measures "d189" distance of L15 L16
  measures "d190" distance of L14 L17
extrude "Extrude20" cut sketch "Sketch20" against normal blind 4 contours L10 L11 L12 L13 bodies 1
copy_body "Body->Comp1" bodies 1 removing the originals makes body 5 in component "body"
sketch "Sketch11 (2)" plane through (0, 0, 30) normal (0, 0, -1) x (1, 0, 0) in component "lid"
  line L0 (41, 17.4) -> (-41.4, 17.4)
  line L1 (-41.4, 17.4) -> (-41.4, 14.4)
  line L2 (-41.4, 14.4) -> (-61, 14.4)
  line L3 (-61, 9) -> (-41, 9)
  line L4 (-41, 9) -> (-41, 5.0657)
  line L5 (-41, 5.0657) -> (-38, 5.0657)
  line L6 (-38, 5.0657) -> (-38, 14)
  line L7 (-38, 14) -> (2, 14)
  line L8 (2, 14) -> (2, 11)
  line L9 (2, 11) -> (4, 11)
  line L10 (4, 11) -> (4, 14)
  line L11 (4, 14) -> (19.5, 14)
  line L12 (19.5, 14) -> (19.5, 15)
  line L13 (19.5, 15) -> (27.5, 15)
  line L14 (27.5, 15) -> (27.5, 14)
  line L15 (27.5, 14) -> (31, 14)
  line L16 (31, 14) -> (31, 11)
  line L17 (31, 11) -> (36.2027, 11)
  line L18 (36.2027, 11) -> (36.2027, -11)
  line L19 (36.2027, -11) -> (31, -11)
  line L20 (31, -11) -> (31, -14)
  line L21 (31, -14) -> (7, -14)
  line L22 (7, -14) -> (7, -11)
  line L23 (7, -11) -> (2, -11)
  line L24 (2, -11) -> (2, -14)
  line L25 (2, -14) -> (-38, -14)
  line L26 (-38, -14) -> (-38, -11)
  line L27 (-38, -11) -> (-39, -11)
  line L28 (-39, -11) -> (-39, -7)
  line L29 (-39, -7) -> (-38, -7)
  line L30 (-38, -7) -> (-38, -5)
  line L31 (-38, -5) -> (-41.0181, -5.0137)
  line L32 (-41.0181, -5.0137) -> (-41, -9)
  line L33 (-41, -9) -> (-61, -9)
  line L34 (-61, -14.4) -> (-41.4, -14.4)
  line L35 (-41.4, -14.4) -> (-41.4, -17.4)
  line L36 (-41.4, -17.4) -> (41, -17.4)
  line L37 (41, -17.4) -> (41, -17)
  line L38 (41, -17) -> (38, -17)
  line L39 (38, -17) -> (38, -14)
  line L40 (38, -14) -> (39, -14)
  line L41 (39, 7) -> (39, 14)
  line L42 (39, 14) -> (38, 14)
  line L43 (38, 14) -> (38, 17)
  line L44 (38, 17) -> (41, 17)
  line L45 (41, 17) -> (41, 17.4)
  line L46 (38, 17) -> (38, 17.4)
  line L47 (38, -17) -> (38, -17.4)
  line L48 (39, -14) -> (39, 7)
  line L49 (-61, 14.4) -> (-61, 9)
  line L50 (-61, -9) -> (-61, -14.4)
  constraint coincident L43.end L44.start
  constraint coincident L0 L46.end
  constraint perpendicular L0 L46
  constraint coincident L38.end L39.start
  constraint coincident L36 L47.end
  constraint perpendicular L36 L47
extrude "Extrude11'" cut sketch "Sketch11 (2)" against normal blind 3 contours L0 L44 L45 L46 | L36 L37 L38 L47 bodies 4 in component "lid"
sketch "Sketch21" plane through (0, -19, 0) normal (0, -1, 0) x (1, 0, 0)
  line L0 (18, 32) -> (18, 30)
  line L1 (18, 30) -> (15, 27)
  line L2 (15, 27) -> (41, 27)
  line L3 (41, 27) -> (41, 32)
  line L4 (41, 32) -> (38, 32)
  line L5 (38, 32) -> (18, 32)
  line L6 (16.051, 27) -> (31.051, 27)
  line L7 (31.051, 27) -> (31.051, 17)
  line L8 (31.051, 17) -> (16.051, 17)
  line L9 (16.051, 17) -> (16.051, 27)
  dimension "d195" = 15
  constraint horizontal L6
  constraint vertical L7
  constraint horizontal L8
  constraint vertical L9
  constraint coincident L2 L6.start
  measures "d195" distance of L6.start L6.end
extrude "Extrude12'" add sketch "Sketch21" against normal up to surface (1.6 mm away) contours L2 L6 L7 L8 L9 bodies 4 in component "lid"
fillet "Fillet3'" radius 1.5 2 edges at (31.051, -18.2, 17) (16.051, -18.2, 17) on bodies 4 in component "lid"
extrude "Extrude14'" cut 1 faces at (38.6667, 14, 31) along direction (0, -1, 0) blind 0.4 on bodies 4 bodies 4 in component "lid"
extrude "Extrude15'" cut 1 faces at (38.3333, -14, 32) along direction (0, 1, 0) blind 0.4 on bodies 4 bodies 4 in component "lid"
chamfer "Chamfer8" distance 0.5 angle 45 4 edges at (39, -13.6, 31.5) (39, -10.3, 33) (39, 3.3, 33) (39, 13.6, 31.5) on bodies 4 in component "lid"
sketch "Sketch12 (2)" plane through (0, -16, 0) normal (0, -1, 0) x (1, 0, 0) in component "lid"
  line L0 (-61, 27) -> (-43, 27)
  line L1 (-43, 27) -> (-43, 32)
  line L2 (-43, 32) -> (-61, 32)
  line L3 (-61, 32) -> (-61, 27)
  line L4 (-61, 33.9028) -> (-54.0972, 27)
  line L5 (-61, 33.9028) -> (-51.238, 33.9028) construction
  line L6 (-61, 33.9028) -> (-61, 27)
  line L7 (-54.0972, 27) -> (-61, 27)
  dimension "d207" = 45
  constraint horizontal L5
  constraint coincident L0 L4.end
  constraint coincident L0.start L3.end
  constraint perpendicular L0 L6
  measures "d207" angle of L4 L5
extrude "Extrude16'" cut sketch "Sketch12 (2)" against normal through all contours L0 L2 L3 L4 L6 L7 | L2 L4 L6 bodies 4 in component "lid"
chamfer "Chamfer1''" distance 11 angle 45 2 edges at (-41, -11.5, 9.5) (-41, 11.5, 9.5) on bodies 5 in component "body"
fillet "Fillet1''" radius 8.5 2 edges at (-54, -11.5, 9.5) (-54, 11.5, 9.5) on bodies 5 in component "body"
component "cam mount" placed x (1, 0, 0) y (0, -1, 0) z (0, 0, -1) at (-56, 0, 18)
component "lid" placed x (1, 0, 0) y (0, 1, 0) z (0, 0, 1) at (0, 0, 0)
component "body" placed x (1, 0, 0) y (0, 1, 0) z (0, 0, 1) at (0, 0, 0)
